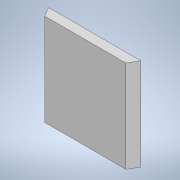
# Autodesk Inventor part: SatelliteSideWallCamera_v2
Saved by Autodesk Inventor 2020 (Build 240168000, 168)
## iProperties
Created: 2020-03-05
Part Number: SatelliteSideWallCamera_v2
Material: Generic
Document SubType Name: Modeling
Designer: WANG
Density: 1 g/cm^3
Appearance: Default
Author: WANG
Autodesk Inventor part; units mm, degrees
ref_plane "YZ Plane" through (0, 0, 0) normal (1, 0, 0) x (0, 1, 0)
ref_plane "XZ Plane" through (0, 0, 0) normal (0, 1, 0) x (-1, 0, 0)
ref_plane "XY Plane" through (0, 0, 0) normal (0, 0, 1) x (1, 0, 0)
sketch "Sketch1" plane through (0, 0, 0) normal (0, 1, 0) x (-1, 0, 0)
  line L0 (-107.95, 0) -> (-53.975, 93.4874)
  line L1 (-53.975, 93.4874) -> (53.975, 93.4874)
  line L2 (53.975, 93.4874) -> (107.95, 0)
  line L3 (107.95, 0) -> (53.975, -93.4874)
  line L4 (53.975, -93.4874) -> (-53.975, -93.4874)
  line L5 (-53.975, -93.4874) -> (-107.95, 0)
  line L6 (-95.25, 0.0344) -> (-47.5952, 82.5062)
  line L7 (-47.5952, 82.5062) -> (47.6548, 82.4717)
  line L8 (47.6548, 82.4717) -> (95.25, -0.0344)
  line L9 (95.25, -0.0344) -> (47.5952, -82.5062)
  line L10 (47.5952, -82.5062) -> (-47.6548, -82.4717)
  line L11 (-47.6548, -82.4717) -> (-95.25, 0.0344)
  line L12 (53.975, -93.4874) -> (47.5952, -82.5062)
  line L13 (-53.975, -93.4874) -> (-47.6548, -82.4717)
  point P0 (0, 0)
  point P1 (0, 0)
  point P2 (0, 0)
  point P3 (0, 0)
  dimension "d0" = 215.9
  dimension "d1" = 12.7
  constraints: 28 end point, 2 coincident, 26 other
  measures "d0" distance of L0.start L2.end
  measures "d1" distance of L0.start L6.start
extrude "Extrusion1" add sketch "Sketch1" along normal blind 107.95 contours L13 L10 L12 L4
body "Solid1"
